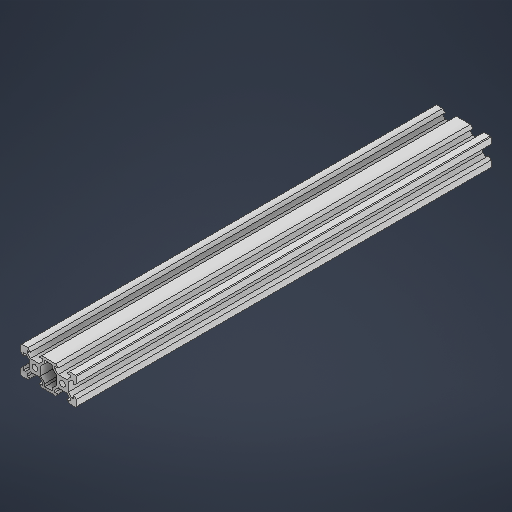
# Autodesk Inventor part: 2040vslot_long
Saved by Autodesk Inventor 2026.1 (Build 301233020, 233B)
## iProperties
Created: 2025-12-18
Part Number: 2040vslot_long
Material: Ogólny
Document SubType Name: Modeling
Designer: maciej
Density: 1 g/cm^3
Appearance: Domyślna
Author: maciej
Autodesk Inventor part; units mm, degrees
ref_plane "YZ Plane" through (0, 0, 0) normal (1, 0, 0) x (0, 1, 0)
ref_plane "XZ Plane" through (0, 0, 0) normal (0, 1, 0) x (-1, 0, 0)
sketch "Szkic1" plane through (0, 0, 0) normal (0, 0, 1) x (1, 0, 0)
  circle A0 centre (0, 0) radius 2.1
  line L0 (-10, 10) -> (10, 10)
  line L1 (10, 10) -> (10, -10)
  line L2 (10, -10) -> (-10, -10)
  line L3 (-10, -10) -> (-10, 10)
  line L4 (-10, -10) -> (10, 10) construction
  line L5 (10, -10) -> (-10, 10) construction
  line L6 (-10, 8.2) -> (10, 8.2)
  line L7 (-10, -8.2) -> (10, -8.2)
  line L8 (-8.2, 10) -> (-8.2, -10)
  line L9 (10, 10) -> (30, 10)
  line L10 (30, 10) -> (30, -10)
  line L11 (30, -10) -> (10, -10)
  line L12 (10, -10) -> (10, 10)
  line L13 (-4.1857, -4.1857) -> (4.1857, -4.1857)
  line L14 (4.1857, -4.1857) -> (4.1857, 4.1857)
  line L15 (4.1857, 4.1857) -> (-4.1857, 4.1857)
  line L16 (-4.1857, 4.1857) -> (-4.1857, -4.1857)
  line L17 (-8.2, 7.1393) -> (-4.1857, 3.125)
  line L18 (-7.1393, 8.2) -> (-3.125, 4.1857)
  line L19 (-4.925, 10) -> (-3.125, 8.2)
  line L20 (4.925, 10) -> (3.125, 8.2)
  line L21 (-3.125, -8.2) -> (-4.925, -10)
  line L22 (3.125, -8.2) -> (4.925, -10)
  line L23 (-8.2, -7.1393) -> (-4.1857, -3.125)
  line L24 (-7.1393, -8.2) -> (-3.125, -4.1857)
  line L25 (3.125, -4.1857) -> (7.1393, -8.2)
  line L26 (4.1857, -3.125) -> (7.3007, -6.24)
  line L27 (4.1857, 3.125) -> (7.3007, 6.24)
  line L28 (3.125, 4.1857) -> (7.1393, 8.2)
  line L29 (-5.4993, 8.2) -> (-5.4993, 6.56)
  line L30 (5.4993, 8.2) -> (5.4993, 6.56)
  line L31 (-8.2, 5.4993) -> (-6.56, 5.4993)
  line L32 (-8.2, -5.4993) -> (-6.56, -5.4993)
  line L33 (-5.4993, -6.56) -> (-5.4993, -8.2)
  line L34 (5.4993, -6.56) -> (5.4993, -8.2)
  line L35 (-8.2, 3.125) -> (-10, 4.925)
  line L36 (-8.2, -3.125) -> (-10, -4.925)
  line L37 (7.3007, 6.24) -> (7.3007, 8.2)
  line L38 (7.3007, -6.24) -> (7.3007, -8.2)
  point P0 (0, -8.2)
  point P1 (-8.2, -8.2)
  point P2 (-8.2, 8.2)
  dimension "d0" = 4.2
  dimension "d1" = 20
  dimension "d2" = 1.8
  dimension "d4" = 20
  dimension "d5" = 20
  dimension "d6" = 1.8
  dimension "d7" = 1.8
  dimension "d8" = 1.5
  dimension "d9" = 0.75
  dimension "d10" = 135
  dimension "d11" = 6.25
  dimension "d12" = 3.125
  dimension "d13" = 1.5
  dimension "d14" = 1.5
  dimension "d15" = 1.5
  dimension "d16" = 0.75
  dimension "d17" = 0.75
  dimension "d18" = 0.75
  dimension "d19" = 1.64
  dimension "d20" = 1.64
  dimension "d21" = 1.64
  dimension "d22" = 1.64
  dimension "d23" = 1.64
  dimension "d24" = 1.64
  dimension "d25" = 45
  dimension "d30" = 1.96
  dimension "d31" = 1.96
  constraints: 74 end point, 35 point on line, 13 perpendicular, 11 parallel, 8 vertical, 4 horizontal, 3 vertical alignment, 2 coincident, 2 horizontal alignment, 1 centre point, 1 midpoint, 21 other
  measures "d0" diameter of A0
  measures "d1" distance of L0.start L0.end
  measures "d2" distance between parallel lines of L3 L8
  measures "d4" distance of L9.end L10.end
  measures "d5" distance between parallel lines of L10 L1
  measures "d8" distance between parallel lines of L18 L17
  measures "d9" distance between parallel lines of L18 L5
  measures "d10" angle of L0 L19
  measures "d11" distance of L22.start L21.start
  measures "d12" distance of L21.start point (0, -8.2)
  measures "d13" distance between parallel lines of L27 L28
  measures "d14" distance between parallel lines of L26 L25
  measures "d15" distance between parallel lines of L23 L24
  measures "d16" distance between parallel lines of L24 L4
  measures "d17" distance between parallel lines of L5 L26
  measures "d18" distance between parallel lines of L28 L4
  measures "d19" distance of L29.start L29.end
  measures "d20" distance of L31.start L31.end
  measures "d21" distance of L33.start L33.end
  measures "d22" distance of L32.start L32.end
  measures "d23" distance of L34.start L34.end
  measures "d24" distance of L30.start L30.end
  measures "d25" angle of L8 L35
  measures "d30" distance of L27.end L37.end
  measures "d31" distance of L26.end L38.end
extrude "Wyciągnięcie proste1" add sketch "Szkic1" along normal blind 300 contours L0 L8 L6 L3 | L0 L19 L6 L8 | L6 L8 L35 L3 | L6 L18 L15 L16 L17 L8 | L0 L1 L6 L20 | L6 L29 L18 | L17 L31 L8 | L36 L8 L7 L3 | L7 L8 L2 L3 | L6 L28 L30 | L15 L14 L13 L16 | L8 L23 L16 L13 L24 L7 | L7 L21 L2 L8 | L32 L23 L8 | L1 L2 L22 L7 | L37 L27 L14 L15 L28 L6 | L24 L33 L7 | L7 L25 L13 L14 L26 L38 | L7 L34 L25
ref_plane "Płaszczyzna konstrukcyjna1" through (10, 8.2, 0) normal (1, 0, 0) x (0, 0, -1)
mirror "Odbij1" about plane through (10, 8.2, 0) normal (1, 0, 0) of "Wyciągnięcie proste1"
fillet "Zaokrąglenie1" radius 0.5 4 edges at (-10, 10, 150) (-10, -10, 150) (30, 10, 150) (30, -10, 150)
